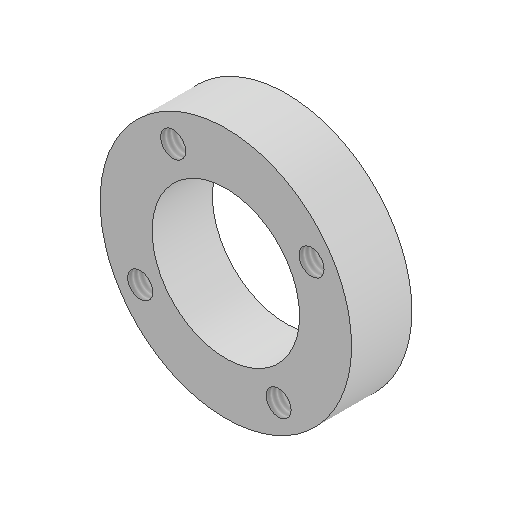
# Autodesk Inventor part: Part16
Saved by Autodesk Inventor 2024 (Build 280153000, 153)
## iProperties
Created: 2023-04-05
Part Number: Part16
Material: Generic
Document SubType Name: Modeling
Designer: ralph
Density: 1 g/cm^3
Appearance: Default
Author: ralph
Autodesk Inventor part; units mm, degrees
ref_plane "YZ Plane" through (0, 0, 0) normal (1, 0, 0) x (0, 1, 0)
ref_plane "XZ Plane" through (0, 0, 0) normal (0, 1, 0) x (-1, 0, 0)
ref_plane "XY Plane" through (0, 0, 0) normal (0, 0, 1) x (1, 0, 0)
sketch "Sketch1" plane through (0, 0, 0) normal (0, 0, 1) x (1, 0, 0)
  circle A0 centre (0, -5) radius 23.8125
  ellipse E0 centre (-25.066556, -29.009567) end of major axis (-17.396721, -26.490299) minor radius 5.878917 (-26.90757, -23.426346) -> (-26.90757, -23.426346) ccw
  line L0 (-26.90757, -23.426346) -> (-27.832023, -23.737709)
  line L1 (-29.265886, -21.408265) -> (-28.524708, -20.677009)
  ellipse E1 centre (-32.727164, -16.564341) end of major axis (-27.02296, -10.851314) minor radius 5.879236 (-28.571485, -20.72316) -> (-28.525164, -20.676548) ccw
  ellipse E2 centre (-32.346551, -17.58951) end of major axis (-24.296384, -18.197133) minor radius 5.879035 (-31.91081, -11.726643) -> (-31.91081, -11.726643) ccw
  line L2 (-31.91081, -11.726643) -> (-32.884047, -11.660532)
  line L3 (-33.317324, -8.95969) -> (-32.352726, -8.567735)
  ellipse E3 centre (-34.661269, -3.160316) end of major axis (-27.205269, -0.065183) minor radius 5.878801 (-32.413603, -8.592472) -> (-32.35297, -8.567134) ccw
  ellipse E4 centre (-34.70212, -4.252716) end of major axis (-41.906987, -0.610674) minor radius 5.879052 (-32.055919, 0.997131) -> (-32.055919, 0.997131) ccw
  line L4 (-32.055919, 0.997131) -> (-32.929773, 1.430651)
  line L5 (-32.296502, 4.091711) -> (-31.255334, 4.084695)
  ellipse E5 centre (-31.318819, 9.963759) end of major axis (-23.246042, 9.970002) minor radius 5.878619 (-31.321044, 4.085138) -> (-31.25533, 4.085343) ccw
  ellipse E6 centre (-31.774878, 8.970095) end of major axis (-37.03772, 15.092271) minor radius 5.879409 (-27.320805, 12.807895) -> (-27.320805, 12.807895) ccw
  line L6 (-27.320805, 12.807895) -> (-27.96224, 13.542826)
  line L7 (-26.35883, 15.758982) -> (-25.399601, 15.354063)
  ellipse E7 centre (-23.208166, 20.81056) end of major axis (-30.669277, 23.894301) minor radius 5.879328 (-25.46014, 15.379618) -> (-25.399349, 15.35466) ccw
  ellipse E8 centre (-24.009591, 20.066548) end of major axis (-26.528865, 27.736399) minor radius 5.878942 (-18.426346, 21.90757) -> (-18.426346, 21.90757) ccw
  line L8 (-18.426346, 21.90757) -> (-18.737709, 22.832023)
  line L9 (-16.408265, 24.265886) -> (-15.677009, 23.524708)
  ellipse E9 centre (-11.564623, 27.726877) end of major axis (-17.277457, 33.430884) minor radius 5.878834 (-15.72316, 23.571485) -> (-15.676548, 23.525164) ccw
  ellipse E10 centre (-12.589421, 27.346544) end of major axis (-11.981802, 35.39665) minor radius 5.878946 (-6.726643, 26.91081) -> (-6.726643, 26.91081) ccw
  line L10 (-6.726643, 26.91081) -> (-6.660532, 27.884047)
  line L11 (-3.95969, 28.317324) -> (-3.567735, 27.352726)
  ellipse E11 centre (1.839847, 29.661337) end of major axis (-1.255331, 37.11745) minor radius 5.878977 (-3.592472, 27.413603) -> (-3.567134, 27.35297) ccw
  ellipse E12 centre (0.747946, 29.701782) end of major axis (4.389762, 36.906192) minor radius 5.878309 (5.997131, 27.055919) -> (5.997131, 27.055919) ccw
  line L12 (5.997131, 27.055919) -> (6.430651, 27.929773)
  line L13 (9.091711, 27.296502) -> (9.084695, 26.255334)
  ellipse E13 centre (14.963894, 26.318821) end of major axis (14.957652, 34.391691) minor radius 5.878755 (9.085138, 26.321044) -> (9.085343, 26.25533) ccw
  ellipse E14 centre (13.970251, 26.774696) end of major axis (20.092302, 32.03743) minor radius 5.87917 (17.807895, 22.320805) -> (17.807895, 22.320805) ccw
  line L14 (17.807895, 22.320805) -> (18.542826, 22.96224)
  line L15 (20.758982, 21.35883) -> (20.354063, 20.399601)
  ellipse E15 centre (25.810277, 18.208281) end of major axis (28.893936, 25.669199) minor radius 5.879023 (20.379618, 20.46014) -> (20.35466, 20.399349) ccw
  ellipse E16 centre (25.066434, 19.009945) end of major axis (32.736527, 21.529301) minor radius 5.879314 (26.90757, 13.426346) -> (26.90757, 13.426346) ccw
  line L16 (26.90757, 13.426346) -> (27.832023, 13.737709)
  line L17 (29.265886, 11.408265) -> (28.524708, 10.677009)
  ellipse E17 centre (32.727281, 6.564224) end of major axis (38.431566, 12.277331) minor radius 5.879402 (28.571485, 10.72316) -> (28.525164, 10.676548) ccw
  ellipse E18 centre (32.346566, 7.5897) end of major axis (40.396864, 6.982068) minor radius 5.879226 (31.91081, 1.726643) -> (31.91081, 1.726643) ccw
  line L18 (31.91081, 1.726643) -> (32.884047, 1.660532)
  line L19 (33.317324, -1.04031) -> (32.352726, -1.432265)
  ellipse E19 centre (34.661448, -6.840109) end of major axis (42.117742, -3.744858) minor radius 5.879261 (32.413603, -1.407528) -> (32.35297, -1.432866) ccw
  ellipse E20 centre (34.701968, -5.747582) end of major axis (27.497307, -2.105643) minor radius 5.878717 (32.055919, -10.997131) -> (32.055919, -10.997131) ccw
  line L20 (32.055919, -10.997131) -> (32.929773, -11.430651)
  line L21 (32.296502, -14.091711) -> (31.255334, -14.084695)
  ellipse E21 centre (31.318824, -19.964675) end of major axis (39.392231, -19.958437) minor radius 5.879535 (31.321044, -14.085138) -> (31.25533, -14.085343) ccw
  ellipse E22 centre (31.774631, -18.970306) end of major axis (26.511936, -12.848298) minor radius 5.879085 (27.320805, -22.807895) -> (27.320805, -22.807895) ccw
  line L22 (27.320805, -22.807895) -> (27.96224, -23.542826)
  line L23 (26.35883, -25.758982) -> (25.399601, -25.354063)
  ellipse E23 centre (23.208233, -30.810396) end of major axis (15.747234, -27.726703) minor radius 5.879151 (25.46014, -25.379618) -> (25.399349, -25.35466) ccw
  ellipse E24 centre (24.00979, -30.066484) end of major axis (21.49047, -22.396496) minor radius 5.879152 (18.426346, -31.90757) -> (18.426346, -31.90757) ccw
  line L24 (18.426346, -31.90757) -> (18.737709, -32.832023)
  line L25 (16.408265, -34.265886) -> (15.677009, -33.524708)
  ellipse E25 centre (11.564423, -37.72708) end of major axis (5.851452, -32.022934) minor radius 5.879119 (15.72316, -33.571485) -> (15.676548, -33.525164) ccw
  ellipse E26 centre (12.58943, -37.346545) end of major axis (13.19705, -29.296433) minor radius 5.878955 (6.726643, -36.91081) -> (6.726643, -36.91081) ccw
  line L26 (6.726643, -36.91081) -> (6.660532, -37.884047)
  line L27 (3.95969, -38.317324) -> (3.567735, -37.352726)
  ellipse E27 centre (-1.840043, -39.66142) end of major axis (-4.935276, -32.205172) minor radius 5.87919 (3.592472, -37.413603) -> (3.567134, -37.35297) ccw
  ellipse E28 centre (-0.747551, -39.701984) end of major axis (2.8944, -32.497302) minor radius 5.878752 (-5.997131, -37.055919) -> (-5.997131, -37.055919) ccw
  line L28 (-5.997131, -37.055919) -> (-6.430651, -37.929773)
  line L29 (-9.091711, -37.296502) -> (-9.084695, -36.255334)
  ellipse E29 centre (-14.964581, -36.318823) end of major axis (-14.970819, -28.245481) minor radius 5.879441 (-9.085138, -36.321044) -> (-9.085343, -36.25533) ccw
  ellipse E30 centre (-13.970405, -36.774515) end of major axis (-7.848476, -31.511889) minor radius 5.878932 (-17.807895, -32.320805) -> (-17.807895, -32.320805) ccw
  line L30 (-17.807895, -32.320805) -> (-18.542826, -32.96224)
  line L31 (-20.758982, -31.35883) -> (-20.354063, -30.399601)
  ellipse E31 centre (-25.810473, -28.208202) end of major axis (-22.726757, -20.74715) minor radius 5.879234 (-20.379618, -30.46014) -> (-20.35466, -30.399349) ccw
  arc A1 (-20.35466, -30.399349) -> (-19.644418, -27.762867) centre (-30.622228, -26.219462) ccw
  arc A2 (-19.644418, -27.762867) -> (-24.163023, -22.894122) centre (-23.857511, -27.141776) ccw
  arc A3 (-24.163023, -22.894122) -> (-26.845089, -23.405986) centre (-23.441695, -33.956404) ccw
  arc A4 (-28.525164, -20.676548) -> (-26.860048, -18.512554) centre (-36.411586, -12.885608) ccw
  arc A5 (-26.860048, -18.512554) -> (-29.171506, -12.285224) centre (-30.514757, -16.32646) ccw
  arc A6 (-29.171506, -12.285224) -> (-31.845294, -11.731743) centre (-32.738439, -22.781481) ccw
  arc A7 (-32.35297, -8.567134) -> (-29.986479, -7.205076) centre (-36.657611, 1.648759) ccw
  arc A8 (-29.986479, -7.205076) -> (-29.738892, -0.567217) centre (-32.526408, -3.786792) ccw
  arc A9 (-29.738892, -0.567217) -> (-31.997342, 0.967347) centre (-37.051052, -8.899488) ccw
  arc A10 (-31.25533, 4.085343) -> (-28.54774, 4.438104) centre (-31.322846, 15.170913) ccw
  arc A11 (-28.54774, 4.438104) -> (-25.778801, 10.475939) centre (-29.586208, 8.568175) ccw
  arc A12 (-25.778801, 10.475939) -> (-27.278084, 12.757962) centre (-35.722978, 5.576167) ccw
  arc A13 (-25.399349, 15.35466) -> (-22.762867, 14.644418) centre (-21.219462, 25.622228) ccw
  arc A14 (-22.762867, 14.644418) -> (-17.894122, 19.163023) centre (-22.141776, 18.857511) ccw
  arc A15 (-17.894122, 19.163023) -> (-18.405986, 21.845089) centre (-28.956404, 18.441695) ccw
  arc A16 (-15.676548, 23.525164) -> (-13.512554, 21.860048) centre (-7.885608, 31.411586) ccw
  arc A17 (-13.512554, 21.860048) -> (-7.285224, 24.171506) centre (-11.32646, 25.514757) ccw
  arc A18 (-7.285224, 24.171506) -> (-6.731743, 26.845294) centre (-17.781481, 27.738439) ccw
  arc A19 (-3.567134, 27.35297) -> (-2.205076, 24.986479) centre (6.648759, 31.657611) ccw
  arc A20 (-2.205076, 24.986479) -> (4.432783, 24.738892) centre (1.213208, 27.526408) ccw
  arc A21 (4.432783, 24.738892) -> (5.967347, 26.997342) centre (-3.899488, 32.051052) ccw
  arc A22 (9.085343, 26.25533) -> (9.438104, 23.54774) centre (20.170913, 26.322846) ccw
  arc A23 (9.438104, 23.54774) -> (15.475939, 20.778801) centre (13.568175, 24.586208) ccw
  arc A24 (15.475939, 20.778801) -> (17.757962, 22.278084) centre (10.576167, 30.722978) ccw
  arc A25 (20.35466, 20.399349) -> (19.644418, 17.762867) centre (30.622228, 16.219462) ccw
  arc A26 (19.644418, 17.762867) -> (24.163023, 12.894122) centre (23.857511, 17.141776) ccw
  arc A27 (24.163023, 12.894122) -> (26.845089, 13.405986) centre (23.441695, 23.956404) ccw
  arc A28 (28.525164, 10.676548) -> (26.860048, 8.512554) centre (36.411586, 2.885608) ccw
  arc A29 (26.860048, 8.512554) -> (29.171506, 2.285224) centre (30.514757, 6.32646) ccw
  arc A30 (29.171506, 2.285224) -> (31.845294, 1.731743) centre (32.738439, 12.781481) ccw
  arc A31 (32.35297, -1.432866) -> (29.986479, -2.794924) centre (36.657611, -11.648759) ccw
  arc A32 (29.986479, -2.794924) -> (29.738892, -9.432783) centre (32.526408, -6.213208) ccw
  arc A33 (29.738892, -9.432783) -> (31.997342, -10.967347) centre (37.051052, -1.100512) ccw
  arc A34 (31.25533, -14.085343) -> (28.54774, -14.438104) centre (31.322846, -25.170913) ccw
  arc A35 (28.54774, -14.438104) -> (25.778801, -20.475939) centre (29.586208, -18.568175) ccw
  arc A36 (25.778801, -20.475939) -> (27.278084, -22.757962) centre (35.722978, -15.576167) ccw
  arc A37 (25.399349, -25.35466) -> (22.762867, -24.644418) centre (21.219462, -35.622228) ccw
  arc A38 (22.762867, -24.644418) -> (17.894122, -29.163023) centre (22.141776, -28.857511) ccw
  arc A39 (17.894122, -29.163023) -> (18.405986, -31.845089) centre (28.956404, -28.441695) ccw
  arc A40 (15.676548, -33.525164) -> (13.512554, -31.860048) centre (7.885608, -41.411586) ccw
  arc A41 (13.512554, -31.860048) -> (7.285224, -34.171506) centre (11.32646, -35.514757) ccw
  arc A42 (7.285224, -34.171506) -> (6.731743, -36.845294) centre (17.781481, -37.738439) ccw
  arc A43 (3.567134, -37.35297) -> (2.205076, -34.986479) centre (-6.648759, -41.657611) ccw
  arc A44 (2.205076, -34.986479) -> (-4.432783, -34.738892) centre (-1.213208, -37.526408) ccw
  arc A45 (-4.432783, -34.738892) -> (-5.967347, -36.997342) centre (3.899488, -42.051052) ccw
  arc A46 (-9.085343, -36.25533) -> (-9.438104, -33.54774) centre (-20.170913, -36.322846) ccw
  arc A47 (-9.438104, -33.54774) -> (-15.475939, -30.778801) centre (-13.568175, -34.586208) ccw
  arc A48 (-15.475939, -30.778801) -> (-17.757962, -32.278084) centre (-10.576167, -40.722978) ccw
  circle A49 centre (0, -5) radius 13.97
  arc A50 (-30.44477, -24.101609) -> (-27.832023, -23.737709) centre (-30.102742, -16.995817) ccw
  arc A51 (-30.767675, -23.57702) -> (-30.44477, -24.101609) centre (0, -5) ccw
  arc A52 (-29.265886, -21.408265) -> (-30.767675, -23.57702) centre (-24.269527, -26.472419) ccw
  arc A53 (-35.437169, -10.996877) -> (-32.884047, -11.660532) centre (-32.401908, -4.562869) ccw
  arc A54 (-35.534743, -10.388649) -> (-35.437169, -10.996877) centre (0, -5) ccw
  arc A55 (-33.317324, -8.95969) -> (-35.534743, -10.388649) centre (-30.639258, -15.550383) ccw
  arc A56 (-35.034581, 3.020825) -> (-32.929773, 1.430651) centre (-29.768177, 7.803529) ccw
  arc A57 (-34.891968, 3.620095) -> (-35.034581, 3.020825) centre (0, -5) ccw
  arc A58 (-32.296502, 4.091711) -> (-34.891968, 3.620095) centre (-32.34444, -3.022146) ccw
  arc A59 (-29.298295, 15.81743) -> (-27.96224, 13.542826) centre (-22.602511, 18.220707) ccw
  arc A60 (-28.937208, 16.316507) -> (-29.298295, 15.81743) centre (0, -5) ccw
  arc A61 (-26.35883, 15.758982) -> (-28.937208, 16.316507) centre (-29.125474, 9.20498) ccw
  arc A62 (-19.101609, 25.44477) -> (-18.737709, 22.832023) centre (-11.995817, 25.102742) ccw
  arc A63 (-18.57702, 25.767675) -> (-19.101609, 25.44477) centre (0, -5) ccw
  arc A64 (-16.408265, 24.265886) -> (-18.57702, 25.767675) centre (-21.472419, 19.269527) ccw
  arc A65 (-5.996877, 30.437169) -> (-6.660532, 27.884047) centre (0.437131, 27.401908) ccw
  arc A66 (-5.388649, 30.534743) -> (-5.996877, 30.437169) centre (0, -5) ccw
  arc A67 (-3.95969, 28.317324) -> (-5.388649, 30.534743) centre (-10.550383, 25.639258) ccw
  arc A68 (8.020825, 30.034581) -> (6.430651, 27.929773) centre (12.803529, 24.768177) ccw
  arc A69 (8.620095, 29.891968) -> (8.020825, 30.034581) centre (0, -5) ccw
  arc A70 (9.091711, 27.296502) -> (8.620095, 29.891968) centre (1.977854, 27.34444) ccw
  arc A71 (20.81743, 24.298295) -> (18.542826, 22.96224) centre (23.220707, 17.602511) ccw
  arc A72 (21.316507, 23.937208) -> (20.81743, 24.298295) centre (0, -5) ccw
  arc A73 (20.758982, 21.35883) -> (21.316507, 23.937208) centre (14.20498, 24.125474) ccw
  arc A74 (30.44477, 14.101609) -> (27.832023, 13.737709) centre (30.102742, 6.995817) ccw
  arc A75 (30.767675, 13.57702) -> (30.44477, 14.101609) centre (0, -5) ccw
  arc A76 (29.265886, 11.408265) -> (30.767675, 13.57702) centre (24.269527, 16.472419) ccw
  arc A77 (35.437169, 0.996877) -> (32.884047, 1.660532) centre (32.401908, -5.437131) ccw
  arc A78 (35.534743, 0.388649) -> (35.437169, 0.996877) centre (0, -5) ccw
  arc A79 (33.317324, -1.04031) -> (35.534743, 0.388649) centre (30.639258, 5.550383) ccw
  arc A80 (35.034581, -13.020825) -> (32.929773, -11.430651) centre (29.768177, -17.803529) ccw
  arc A81 (34.891968, -13.620095) -> (35.034581, -13.020825) centre (0, -5) ccw
  arc A82 (32.296502, -14.091711) -> (34.891968, -13.620095) centre (32.34444, -6.977854) ccw
  arc A83 (29.298295, -25.81743) -> (27.96224, -23.542826) centre (22.602511, -28.220707) ccw
  arc A84 (28.937208, -26.316507) -> (29.298295, -25.81743) centre (0, -5) ccw
  arc A85 (26.35883, -25.758982) -> (28.937208, -26.316507) centre (29.125474, -19.20498) ccw
  arc A86 (19.101609, -35.44477) -> (18.737709, -32.832023) centre (11.995817, -35.102742) ccw
  arc A87 (18.57702, -35.767675) -> (19.101609, -35.44477) centre (0, -5) ccw
  arc A88 (16.408265, -34.265886) -> (18.57702, -35.767675) centre (21.472419, -29.269527) ccw
  arc A89 (5.996877, -40.437169) -> (6.660532, -37.884047) centre (-0.437131, -37.401908) ccw
  arc A90 (5.388649, -40.534743) -> (5.996877, -40.437169) centre (0, -5) ccw
  arc A91 (3.95969, -38.317324) -> (5.388649, -40.534743) centre (10.550383, -35.639258) ccw
  arc A92 (-8.020825, -40.034581) -> (-6.430651, -37.929773) centre (-12.803529, -34.768177) ccw
  arc A93 (-8.620095, -39.891968) -> (-8.020825, -40.034581) centre (0, -5) ccw
  arc A94 (-9.091711, -37.296502) -> (-8.620095, -39.891968) centre (-1.977854, -37.34444) ccw
  arc A95 (-20.81743, -34.298295) -> (-18.542826, -32.96224) centre (-23.220707, -27.602511) ccw
  arc A96 (-21.316507, -33.937208) -> (-20.81743, -34.298295) centre (0, -5) ccw
  arc A97 (-20.758982, -31.35883) -> (-21.316507, -33.937208) centre (-14.20498, -34.125474) ccw
  circle A98 centre (16.222975, 4.985869) radius 2.38125
  circle A99 centre (9.985869, -21.222975) radius 2.38125
  circle A100 centre (-9.985869, 11.222975) radius 2.38125
  circle A101 centre (-16.222975, -14.985869) radius 2.38125
  point P0 (0, 0)
  dimension "d0" = 47.625
  constraints: 1 centre point, 32 other
  measures "d0" diameter of A0
sketch "Sketch1 outline for Extrusion1" plane through (0, 0, 0) normal (0, 0, 1) x (1, 0, 0)
  circle A0 centre (0, -5) radius 23.8125
extrude "Extrusion1" add sketch "Sketch1 outline for Extrusion1" along normal blind 9.525
sketch "Sketch2" plane through (0, -5, 9.525) normal (0, 0, 1) x (1, 0, 0)
  circle A0 centre (0, 0) radius 13.97
  point P0 (0, 5)
  dimension "d3" = 27.94
  constraints: 1 centre point
  measures "d3" diameter of A0
extrude "Extrusion2" cut sketch "Sketch2" against normal blind 26.9875
sketch "Sketch3" plane through (0, -5, 9.525) normal (0, 0, 1) x (1, 0, 0)
  circle A0 centre (0, 0) radius 13.97 projected
  circle A1 centre (0, 0) radius 23.8125 projected
  point P0 (0, 5)
extrude "Extrusion3" add sketch "Sketch3" against normal blind 11.43
sketch "Sketch4" plane through (0, -5, 9.525) normal (0, 0, 1) x (1, 0, 0)
  circle A0 centre (16.222975, 9.985869) radius 2.38125
  circle A1 centre (9.985869, -16.222975) radius 2.38125
  circle A2 centre (-9.985869, 16.222975) radius 2.38125
  circle A3 centre (-16.222975, -9.985869) radius 2.38125
  circle A4 centre (0, 0) radius 13.97
  arc A5 (32.35297, 3.567134) -> (31.845294, 6.731743) centre (0, 0) ccw
  arc A6 (29.171506, 7.285224) -> (31.845294, 6.731743) centre (32.738439, 17.781481) ccw
  arc A7 (26.860048, 13.512554) -> (29.171506, 7.285224) centre (30.514757, 11.32646) ccw
  arc A8 (28.525164, 15.676548) -> (26.860048, 13.512554) centre (36.411586, 7.885608) ccw
  arc A9 (28.525164, 15.676548) -> (26.845089, 18.405986) centre (0, 0) ccw
  arc A10 (24.163023, 17.894122) -> (26.845089, 18.405986) centre (23.441695, 28.956404) ccw
  arc A11 (19.644418, 22.762867) -> (24.163023, 17.894122) centre (23.857511, 22.141776) ccw
  arc A12 (20.35466, 25.399349) -> (19.644418, 22.762867) centre (30.622228, 21.219462) ccw
  arc A13 (20.35466, 25.399349) -> (17.757962, 27.278084) centre (0, 0) ccw
  arc A14 (15.475939, 25.778801) -> (17.757962, 27.278084) centre (10.576167, 35.722978) ccw
  arc A15 (9.438104, 28.54774) -> (15.475939, 25.778801) centre (13.568175, 29.586208) ccw
  arc A16 (9.085343, 31.25533) -> (9.438104, 28.54774) centre (20.170913, 31.322846) ccw
  arc A17 (9.085343, 31.25533) -> (5.967347, 31.997342) centre (0, 0) ccw
  arc A18 (4.432783, 29.738892) -> (5.967347, 31.997342) centre (-3.899488, 37.051052) ccw
  arc A19 (-2.205076, 29.986479) -> (4.432783, 29.738892) centre (1.213208, 32.526408) ccw
  arc A20 (-3.567134, 32.35297) -> (-2.205076, 29.986479) centre (6.648759, 36.657611) ccw
  arc A21 (-3.567134, 32.35297) -> (-6.731743, 31.845294) centre (0, 0) ccw
  arc A22 (-7.285224, 29.171506) -> (-6.731743, 31.845294) centre (-17.781481, 32.738439) ccw
  arc A23 (-13.512554, 26.860048) -> (-7.285224, 29.171506) centre (-11.32646, 30.514757) ccw
  arc A24 (-15.676548, 28.525164) -> (-13.512554, 26.860048) centre (-7.885608, 36.411586) ccw
  arc A25 (-15.676548, 28.525164) -> (-18.405986, 26.845089) centre (0, 0) ccw
  arc A26 (-17.894122, 24.163023) -> (-18.405986, 26.845089) centre (-28.956404, 23.441695) ccw
  arc A27 (-22.762867, 19.644418) -> (-17.894122, 24.163023) centre (-22.141776, 23.857511) ccw
  arc A28 (-25.399349, 20.35466) -> (-22.762867, 19.644418) centre (-21.219462, 30.622228) ccw
  arc A29 (-25.399349, 20.35466) -> (-27.278084, 17.757962) centre (0, 0) ccw
  arc A30 (-25.778801, 15.475939) -> (-27.278084, 17.757962) centre (-35.722978, 10.576167) ccw
  arc A31 (-28.54774, 9.438104) -> (-25.778801, 15.475939) centre (-29.586208, 13.568175) ccw
  arc A32 (-31.25533, 9.085343) -> (-28.54774, 9.438104) centre (-31.322846, 20.170913) ccw
  arc A33 (-31.25533, 9.085343) -> (-31.997342, 5.967347) centre (0, 0) ccw
  arc A34 (-29.738892, 4.432783) -> (-31.997342, 5.967347) centre (-37.051052, -3.899488) ccw
  arc A35 (-29.986479, -2.205076) -> (-29.738892, 4.432783) centre (-32.526408, 1.213208) ccw
  arc A36 (-32.35297, -3.567134) -> (-29.986479, -2.205076) centre (-36.657611, 6.648759) ccw
  arc A37 (-32.35297, -3.567134) -> (-31.845294, -6.731743) centre (0, 0) ccw
  arc A38 (-29.171506, -7.285224) -> (-31.845294, -6.731743) centre (-32.738439, -17.781481) ccw
  arc A39 (-26.860048, -13.512554) -> (-29.171506, -7.285224) centre (-30.514757, -11.32646) ccw
  arc A40 (-28.525164, -15.676548) -> (-26.860048, -13.512554) centre (-36.411586, -7.885608) ccw
  arc A41 (-28.525164, -15.676548) -> (-26.845089, -18.405986) centre (0, 0) ccw
  arc A42 (-24.163023, -17.894122) -> (-26.845089, -18.405986) centre (-23.441695, -28.956404) ccw
  arc A43 (-19.644418, -22.762867) -> (-24.163023, -17.894122) centre (-23.857511, -22.141776) ccw
  arc A44 (-20.35466, -25.399349) -> (-19.644418, -22.762867) centre (-30.622228, -21.219462) ccw
  arc A45 (-20.35466, -25.399349) -> (-17.757962, -27.278084) centre (0, 0) ccw
  arc A46 (-15.475939, -25.778801) -> (-17.757962, -27.278084) centre (-10.576167, -35.722978) ccw
  arc A47 (-9.438104, -28.54774) -> (-15.475939, -25.778801) centre (-13.568175, -29.586208) ccw
  arc A48 (-9.085343, -31.25533) -> (-9.438104, -28.54774) centre (-20.170913, -31.322846) ccw
  arc A49 (-9.085343, -31.25533) -> (-5.967347, -31.997342) centre (0, 0) ccw
  arc A50 (-4.432783, -29.738892) -> (-5.967347, -31.997342) centre (3.899488, -37.051052) ccw
  arc A51 (2.205076, -29.986479) -> (-4.432783, -29.738892) centre (-1.213208, -32.526408) ccw
  arc A52 (3.567134, -32.35297) -> (2.205076, -29.986479) centre (-6.648759, -36.657611) ccw
  arc A53 (3.567134, -32.35297) -> (6.731743, -31.845294) centre (0, 0) ccw
  arc A54 (7.285224, -29.171506) -> (6.731743, -31.845294) centre (17.781481, -32.738439) ccw
  arc A55 (13.512554, -26.860048) -> (7.285224, -29.171506) centre (11.32646, -30.514757) ccw
  arc A56 (15.676548, -28.525164) -> (13.512554, -26.860048) centre (7.885608, -36.411586) ccw
  arc A57 (15.676548, -28.525164) -> (18.405986, -26.845089) centre (0, 0) ccw
  arc A58 (17.894122, -24.163023) -> (18.405986, -26.845089) centre (28.956404, -23.441695) ccw
  arc A59 (22.762867, -19.644418) -> (17.894122, -24.163023) centre (22.141776, -23.857511) ccw
  arc A60 (25.399349, -20.35466) -> (22.762867, -19.644418) centre (21.219462, -30.622228) ccw
  arc A61 (25.399349, -20.35466) -> (27.278084, -17.757962) centre (0, 0) ccw
  arc A62 (25.778801, -15.475939) -> (27.278084, -17.757962) centre (35.722978, -10.576167) ccw
  arc A63 (28.54774, -9.438104) -> (25.778801, -15.475939) centre (29.586208, -13.568175) ccw
  arc A64 (31.25533, -9.085343) -> (28.54774, -9.438104) centre (31.322846, -20.170913) ccw
  arc A65 (31.25533, -9.085343) -> (31.997342, -5.967347) centre (0, 0) ccw
  arc A66 (29.738892, -4.432783) -> (31.997342, -5.967347) centre (37.051052, 3.899488) ccw
  arc A67 (29.986479, 2.205076) -> (29.738892, -4.432783) centre (32.526408, -1.213208) ccw
  arc A68 (32.35297, 3.567134) -> (29.986479, 2.205076) centre (36.657611, -6.648759) ccw
  point P0 (0, 5)
extrude "Extrusion4" cut sketch "Sketch4" against normal blind 11.43 contours A0 | A1 | A2 | A3
thread "Thread1" size "10-24 UNC" class "2B" standard "ANSI Unified Screw Threads" full length
thread "Thread2" size "10-24 UNC" class "2B" standard "ANSI Unified Screw Threads" full length
thread "Thread3" size "10-24 UNC" class "2B" standard "ANSI Unified Screw Threads" full length
thread "Thread4" size "10-24 UNC" class "2B" standard "ANSI Unified Screw Threads" full length
body "Solid1"
